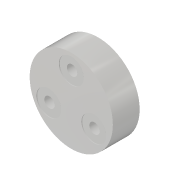
# Autodesk Inventor part: membrane_mold
Saved by Autodesk Inventor 2018 (Build 220112000, 112)
## iProperties
Created: 2019-06-14
Part Number: membrane_mold
Material: Generic
Document SubType Name: Modeling
Designer: amink
Density: 1 g/cm^3
Appearance: Default
Author: amink
Autodesk Inventor part; units mm, degrees
ref_plane "YZ Plane" through (0, 0, 0) normal (1, 0, 0) x (0, 1, 0)
ref_plane "XZ Plane" through (0, 0, 0) normal (0, 1, 0) x (-1, 0, 0)
ref_plane "XY Plane" through (0, 0, 0) normal (0, 0, 1) x (1, 0, 0)
sketch "Sketch1" plane through (0, 0, 0) normal (0, 0, 1) x (1, 0, 0)
  circle A0 centre (0, 0) radius 101.6
  dimension "d10" = 203.2
  constraints: 1 centre point, 1 coincident
  measures "d10" diameter of A0
extrude "Extrusion1" add sketch "Sketch1" along normal blind 90
sketch "Sketch2" plane through (0, 0, 90) normal (0, 0, 1) x (1, 0, 0)
  circle A0 centre (0, 63.5) radius 30.226
  circle A1 centre (-54.9926, -31.75) radius 30.226
  circle A2 centre (54.9926, -31.75) radius 30.226
  point P0 (0, 0)
  dimension "d4" = 360
  dimension "d11" = 63.5
  dimension "d12" = 60.452
  constraints: 3 centre point, 7 other
  measures "d11" distance of point (0, 0) A0.centre
  measures "d12" diameter of A0
extrude "Extrusion2" cut sketch "Sketch2" against normal blind 2
sketch "Sketch5" plane through (0, 0, 0) normal (0, 0, -1) x (-1, 0, 0)
  circle A0 centre (0, 0) radius 88.9
  dimension "d13" = 177.8
  constraints: 1 centre point, 1 coincident
  measures "d13" diameter of A0
extrude "Extrusion4" add sketch "Sketch5" along normal blind 1.5
sketch "Sketch6" plane through (0, 0, 90) normal (0, 0, 1) x (1, 0, 0)
  circle A0 centre (54.9926, -31.75) radius 30.226 projected
  circle A1 centre (54.9926, -31.75) radius 12.7
  circle A2 centre (0, 63.5) radius 12.7
  circle A3 centre (-54.9926, -31.75) radius 12.7
  point P0 (0, 0)
  dimension "d16" = 25.4
  dimension "d19" = 360
  constraints: 3 centre point, 1 coincident, 7 other
  measures "d16" diameter of A1
extrude "Extrusion5" cut sketch "Sketch6" against normal blind 53.8 contours A1 | A2 | A3
body "Solid1"
